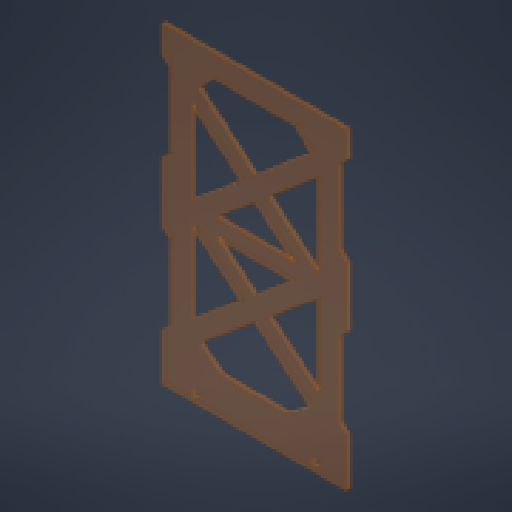
# Autodesk Inventor part: Shelf1
Saved by Autodesk Inventor 2023.4 (Build 274418000, 418)
## iProperties
Created: 2025-10-22
Part Number: Shelf1
Material: Generic
Document SubType Name: Modeling
Designer: Malthe Sennels
Density: 1 g/cm^3
Appearance: Polycarbonate - Clear
Author: Malthe Sennels
Autodesk Inventor part; units mm, degrees
ref_plane "YZ Plane" through (0, 0, 0) normal (1, 0, 0) x (0, 1, 0)
ref_plane "XZ Plane" through (0, 0, 0) normal (0, 1, 0) x (-1, 0, 0)
ref_plane "XY Plane" through (0, 0, 0) normal (0, 0, 1) x (1, 0, 0)
sketch "Sketch1" plane through (0, 0, 0) normal (0, 0, 1) x (1, 0, 0)
  line L0 (-120, 25) -> (-122, 25) construction
  line L1 (-122, 0) -> (-122, 25) projected
  line L2 (-110, 0) -> (-122, 0) projected
  line L3 (-120, 10) -> (-110, 0) construction
  line L4 (-120, 10) -> (-120, 18.3797) construction
  line L5 (-80.5845, 0) -> (-120, 18.3797) construction
  line L6 (-66.3873, 0) -> (-80.5845, 0) projected
  line L7 (-120, 25) -> (-66.3873, 0) construction
  line L8 (2, 25) -> (0, 25) construction
  line L9 (-53.6127, 0) -> (0, 25) construction
  line L10 (-39.4155, 0) -> (-53.6127, 0) projected
  line L11 (0, 18.3797) -> (-39.4155, 0) construction
  line L12 (0, 10) -> (0, 18.3797) construction
  line L13 (-10, 0) -> (0, 10) construction
  line L14 (2, 0) -> (-10, 0) projected
  line L15 (2, 0) -> (2, 25) projected
  line L16 (2, 0) -> (-122, 0)
  line L17 (-122, 0) -> (-122, 210)
  line L18 (-122, 210) -> (2, 210)
  line L19 (2, 210) -> (2, 0)
  circle A0 centre (-100, 5) radius 2.25 projected
  circle A1 centre (-20, 5) radius 2.25 projected
  line L20 (2, 32) -> (-3, 37)
  line L21 (2, 32) -> (9.0711, 32) construction
  line L22 (-3, 37) -> (-3, 87)
  line L23 (-3, 87) -> (2, 92)
  line L24 (2, 132) -> (-3, 137)
  line L25 (2, 132) -> (9.0711, 132) construction
  line L26 (-3, 137) -> (-3, 187)
  line L27 (-3, 187) -> (2, 192)
  line L28 (-60, 0) -> (-60, 210) construction
  line L29 (-122, 32) -> (-117, 37)
  line L30 (-122, 32) -> (-129.0711, 32) construction
  line L31 (-117, 37) -> (-117, 87)
  line L32 (-117, 87) -> (-122, 92)
  line L33 (-122, 132) -> (-117, 137)
  line L34 (-122, 132) -> (-129.0711, 132) construction
  line L35 (-117, 137) -> (-117, 187)
  line L36 (-117, 187) -> (-122, 192)
  line L37 (-38, 25) -> (-18, 40)
  line L38 (2, 200.3422) -> (-7.6578, 210)
  line L39 (-38, 25) -> (-60, 25)
  line L40 (-18, 40) -> (-18, 180)
  line L41 (-18, 40) -> (122, 40) construction
  line L42 (-18, 180) -> (-33, 195)
  line L43 (-33, 195) -> (-60, 195)
  line L44 (-82, 25) -> (-102, 40)
  line L45 (-82, 25) -> (-60, 25)
  line L46 (-102, 40) -> (-102, 180)
  line L47 (-102, 180) -> (-87, 195)
  line L48 (-87, 195) -> (-60, 195)
  line L49 (-122, 200.3422) -> (-112.3422, 210)
  line L50 (-18, 40) -> (-102, 109.2728)
  line L51 (-18, 109.2728) -> (-102, 109.2728)
  line L52 (-102, 40) -> (-18, 109.2728)
  line L53 (-18, 109.2728) -> (-102, 180)
  line L54 (-102, 109.2728) -> (-18, 180)
  line L55 (-98.1826, 35.371) -> (-14.1826, 104.6439)
  line L56 (-105.8174, 44.629) -> (-21.8174, 113.9018)
  line L57 (-14.1826, 44.629) -> (-98.1826, 113.9018)
  line L58 (-21.8174, 35.371) -> (-105.8174, 104.6439)
  line L59 (-98.1355, 104.6831) -> (-14.1355, 175.4103)
  line L60 (-105.8645, 113.8626) -> (-21.8645, 184.5897)
  line L61 (-21.8645, 104.6831) -> (-105.8645, 175.4103)
  line L62 (-14.1355, 113.8626) -> (-98.1355, 184.5897)
  line L63 (-18, 103.2728) -> (-102, 103.2728)
  line L64 (-18, 115.2728) -> (-102, 115.2728)
  point P0 (0, 0)
  point P1 (2, 25)
  point P2 (-60, 66.8593)
  point P3 (-22.9389, 36.2959)
  point P4 (-97.0611, 36.2959)
  point P5 (-69.4305, 74.6364)
  point P6 (-102, 47.7771)
  point P7 (-102, 101.4957)
  point P8 (-34.7061, 103.2728)
  point P9 (-60, 82.4135)
  point P10 (-85.2939, 103.2728)
  point P11 (-50.5695, 74.6364)
  point P12 (-18, 101.4957)
  point P13 (-18, 47.7771)
  point P14 (-69.3156, 144.6364)
  point P15 (-102, 117.1164)
  point P16 (-102, 172.1564)
  point P17 (-50.6844, 144.6364)
  point P18 (-18, 172.1564)
  point P19 (-18, 117.1164)
  point P20 (-60, 152.48)
  point P21 (-97.7418, 184.2582)
  point P22 (-22.2582, 184.2582)
  point P23 (-85.5585, 115.2728)
  point P24 (-60, 136.7928)
  point P25 (-34.4415, 115.2728)
  dimension "d0" = 124
  dimension "d1" = 210
  dimension "d4" = 135
  dimension "d5" = 5
  dimension "d6" = 60
  dimension "d7" = 135
  dimension "d8" = 60
  dimension "d9" = 40
  dimension "d10" = 32
  dimension "d11" = 5
  dimension "d12" = 90
  dimension "d13" = 135
  dimension "d14" = 15
  dimension "d15" = 25
  dimension "d16" = 40
  dimension "d17" = 15
  dimension "d18" = 15
  dimension "d19" = 20
  dimension "d20" = 6
  dimension "d21" = 6
  dimension "d22" = 6
  dimension "d23" = 6
  dimension "d24" = 6
  dimension "d25" = 6
  dimension "d26" = 6
  dimension "d27" = 6
  dimension "d28" = 6
  dimension "d29" = 6
  constraints: 98 end point, 16 symmetric about line, 12 parallel, 10 point on line, 6 perpendicular, 5 horizontal, 3 equal length, 2 midpoint, 2 vertical
  measures "d0" distance of L17.end L18.end
  measures "d1" distance from line of L2.start L18
  measures "d4" angle of L21 L20
  measures "d5" distance between parallel lines of L19 L22
  measures "d6" distance of L20.start L23.end
  measures "d7" angle of L25 L24
  measures "d8" distance of L24.start L27.end
  measures "d9" distance of L23.end L24.start
  measures "d10" distance of L14.start L20.start
  measures "d11" distance between parallel lines of L19 L26
  measures "d12" angle of L41 L40
  measures "d13" angle of L42 L40
  measures "d14" distance between parallel lines of L43 L18
  measures "d15" distance between parallel lines of L16 L39
  measures "d16" distance from line of L16 L37.end
  measures "d17" distance from line of L26 L40.end
  measures "d18" horizontal distance of L40.end L42.end
  measures "d19" horizontal distance of L37.start L37.end
  measures "d20" distance between parallel lines of L52 L55
  measures "d21" distance between parallel lines of L52 L56
  measures "d22" distance between parallel lines of L50 L57
  measures "d23" distance between parallel lines of L50 L58
  measures "d24" distance between parallel lines of L54 L59
  measures "d25" distance between parallel lines of L54 L60
  measures "d26" distance between parallel lines of L53 L61
  measures "d27" distance between parallel lines of L53 L62
  measures "d28" distance between parallel lines of L51 L63
  measures "d29" distance between parallel lines of L51 L64
extrude "Extrusion1" add sketch "Sketch1" along normal blind 3 contours L1 L17 L29 L31 L32 L33 L35 L36 L49 L18 L38 L19 L27 L26 L24 L23 L22 L20 L15 L14 L16 L10 L6 L2 | L58 L55 L50 L37 | L50 L55 L57 L40 | L58 L52 L50 L55 | L55 L44 L52 L58 | L50 L52 L57 L55 | L58 L56 L50 L52 | L52 L46 L56 L58 | L55 L57 L52 L63 L40 | L50 L56 L57 L52 | L58 L46 L63 L50 L56 | L63 L52 L40 | L57 L56 L63 L52 | L50 L63 L57 L56 | L53 L64 L40 | L52 L61 L51 | L51 L61 L56 L53 | L63 L56 L51 L61 L52 | L63 L46 L50 | L50 L59 L51 L57 L63 | L64 L53 L59 L62 L40 | L51 L56 L61 | L56 L61 L64 L53 | L63 L57 L51 L56 | L50 L51 L59 | L54 L57 L59 L51 | L46 L64 L54 | L64 L61 L59 L53 | L51 L57 L59 L64 L61 L56 | L51 L59 L57 | L46 L60 L61 L54 L64 | L54 L64 L59 L57 | L59 L62 L54 L40 | L59 L53 L54 L62 | L59 L61 L54 L53 | L54 L61 L59 L64 | L54 L62 L60 L42 | L54 L53 L60 L62 | L54 L61 L60 L53 | L46 L53 L60 L61 | L60 L53 L47 L62
body "Solid1"
